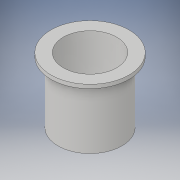
# Autodesk Inventor part: Carrier
Saved by Autodesk Inventor 2017 (Build 210142000, 142)
## iProperties
Created: 2016-07-19
Part Number: Carrier
Material: Generic
Document SubType Name: Modeling
Designer: Bill
Density: 1 g/cm^3
Appearance: Default
Author: Bill
Autodesk Inventor part; units mm, degrees
ref_plane "YZ Plane" through (0, 0, 0) normal (1, 0, 0) x (0, 1, 0)
ref_plane "XZ Plane" through (0, 0, 0) normal (0, 1, 0) x (-1, 0, 0)
ref_plane "XY Plane" through (0, 0, 0) normal (0, 0, 1) x (1, 0, 0)
sketch "Sketch1" plane through (0, 0, 0) normal (0, 0, 1) x (1, 0, 0)
  line L0 (-80.0608, -33.7915) -> (-73.7108, -33.7915)
  line L1 (-73.7108, -33.7915) -> (-60.5784, 15.2194)
  line L2 (-60.5784, 15.2194) -> (-66.9284, 15.2194)
  line L3 (-66.9284, 15.2194) -> (-66.9284, 129.5194)
  line L4 (-66.9284, 129.5194) -> (-97.9932, 129.5194)
  line L5 (-97.9932, 129.5194) -> (-97.9932, 119.9944)
  line L6 (-97.9932, 119.9944) -> (-80.0608, 119.9944)
  line L7 (-80.0608, 119.9944) -> (-80.0608, -33.7915)
  line L8 (0, -66.4537) -> (0, 162.1816) projected
  point P0 (0, 0)
  dimension "d0" = 6.35
  dimension "d1" = 105
  dimension "d2" = 6.35
  dimension "d3" = 114.3
  dimension "d4" = 73.7108
  dimension "d6" = 9.525
  dimension "d8" = 17.9324
  dimension "d10" = 60.5784
  constraints: 16 end point, 5 perpendicular, 1 horizontal, 1 parallel
  measures "d0" distance of L0.start L0.end
  measures "d1" angle of L0 L1
  measures "d2" distance of L1.end L2.end
  measures "d3" distance of L2.end L3.end
  measures "d4" horizontal distance of point (0, 0) L0.end
  measures "d6" distance of L4.end L5.end
  measures "d8" distance of L5.end L6.end
  measures "d10" distance from line of L8 L1.end
revolve "Revolution1" add sketch "Sketch1" angle 360 about axis through (0, -10, 0) along (0, 1, 0)
body "Solid1"
